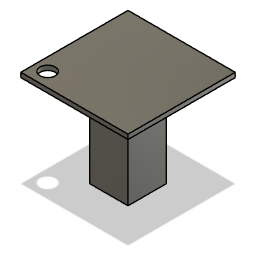
Gps mount v2 (Autodesk Fusion 360 design; units mm, degrees)
Autodesk Fusion 360 part; units mm, degrees
sketch "Sketch1" plane through (0, 0, 0) normal (0, 1, 0) x (1, 0, 0)
  line L0 (0, 0) -> (25, 0)
  line L1 (25, 0) -> (25, -25)
  line L2 (25, -25) -> (0, -25)
  line L3 (0, -25) -> (0, 0)
  dimension "d1" = 25
  dimension "d2" = 25
  constraint horizontal L0
  constraint vertical L1
  constraint horizontal L2
  constraint vertical L3
  constraint coincident L0.start L3.end
  measures "d1" distance of L0.start L0.end
  measures "d2" distance of L0.start L2.end
extrude "Extrude1" add sketch "Sketch1" along normal blind 60
sketch "Sketch2" plane through (0, 60, 0) normal (0, 1, 0) x (-1, 0, 0)
  line L0 (0, 25) -> (-25, 25)
  line L1 (-25, 25) -> (-25, 0)
  line L2 (-25, 0) -> (0, 0)
  line L3 (0, 0) -> (0, 25)
  line L4 (-47.5, 47.5) -> (22.5, 47.5)
  line L5 (22.5, 47.5) -> (22.5, -22.5)
  line L6 (22.5, -22.5) -> (-47.5, -22.5)
  line L7 (-47.5, -22.5) -> (-47.5, 47.5)
  line L8 (-47.5, 47.5) -> (22.5, -22.5) construction
  line L9 (22.5, 47.5) -> (-47.5, -22.5) construction
  point P0 (-12.5, 12.5)
  dimension "d5" = 70
  dimension "d6" = 70
  constraint horizontal L4
  constraint perpendicular L4 L5
  constraint parallel L4 L6
  constraint parallel L5 L7
  constraint coincident L8 P0
  constraint coincident L9 P0
  measures "d5" distance of L5.end L6.end
  measures "d6" distance of L4.end L5.end
extrude "Extrude2" add sketch "Sketch2" along normal blind 3 contours L0 L1 L2 L3 | L4 L5 L6 L7
fillet "Fillet1" radius 10 4 edges at (12.5, 60, 25) (25, 60, 12.5) (0, 60, 12.5) (12.5, 60, 0)
sketch "Sketch3" plane through (0, 63, 0) normal (0, 1, 0) x (-1, 0, 0)
  line L0 (-47.5, -22.5) -> (22.5, -22.5)
  line L1 (22.5, -22.5) -> (22.5, 47.5)
  line L2 (22.5, 47.5) -> (-47.5, 47.5)
  line L3 (-47.5, 47.5) -> (-47.5, -22.5)
  circle A0 centre (14.2428, 38.2388) radius 5
  dimension "d11" = 10
  measures "d11" diameter of A0
extrude "Extrude3" cut sketch "Sketch3" against normal blind 30 contours A0
sketch "Sketch4" plane through (0, 0, 0) normal (0, 1, 0) x (1, 0, 0)
  line L0 (25, 0) -> (0, 0)
  line L1 (0, 0) -> (0, -25)
  line L2 (0, -25) -> (25, -25)
  line L3 (25, -25) -> (25, 0)
  circle A0 centre (18.75, -6.25) radius 1.5
  circle A1 centre (18.767, -18.75) radius 1.5
  circle A2 centre (6.25, -6.25) radius 1.5
  circle A3 centre (6.233, -18.75) radius 1.5
  point P0 (25, 0)
  point P1 (25, -25)
  dimension "d14" = 3
  dimension "d15" = 3
  dimension "d17" = 12.5
  dimension "d18" = 6.25
  constraint horizontal L0
  constraint vertical L1
  constraint horizontal L2
  constraint vertical L3
  constraint coincident L0 P0
  constraint coincident L2 P1
  measures "d14" diameter of A0
  measures "d15" diameter of A1
  measures "d17" vertical distance of A0.centre A1.centre
  measures "d18" distance of L2 A1.centre
extrude "Extrude4" cut sketch "Sketch4" along normal blind 7 contours A0 | A1 | A2 | A3
equation "d17 = 2.5 / 2 * 1 cm"
equation "d18 = 2.5 / 4 * 1 cm"
